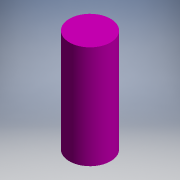
# Autodesk Inventor part: Connector
Saved by Autodesk Inventor 2017 (Build 210142000, 142)
## iProperties
Part Number: Connector
Material: Generic
Document SubType Name: Modeling
Designer: Alexander Miller
Appearance: Magenta
Author: Alexander Miller
Autodesk Inventor part; units mm, degrees
ref_plane "YZ Plane" through (0, 0, 0) normal (1, 0, 0) x (0, 1, 0)
ref_plane "XZ Plane" through (0, 0, 0) normal (0, 1, 0) x (-1, 0, 0)
ref_plane "XY Plane" through (0, 0, 0) normal (0, 0, 1) x (1, 0, 0)
sketch "Sketch1" plane through (0, 0, 0) normal (0, 1, 0) x (-1, 0, 0)
  circle A0 centre (0, 0) radius 2
  dimension "d0" = 4
  constraints: 1 centre point, 1 coincident
  measures "d0" diameter of A0
extrude "Extrusion1" add sketch "Sketch1" along normal blind 10
equation "\"d0\" = bb_inner_diameter"
equation "\"d1\" = 2 * b_mat_thickness"
equation "\"bb_inner_diameter\" = 4"
equation "\"b_mat_thickness\" = 5"
body "Solid1"
